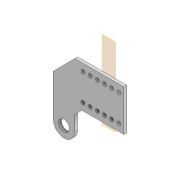
# Autodesk Inventor part: driven wheel arm angled adjustable holes
Saved by Autodesk Inventor 2020 (Build 240168000, 168)
## iProperties
Created: 2020-01-25
Part Number: driven wheel arm angled adjustable holes
Material: Generic
Document SubType Name: Modeling
Designer: ball
Density: 1 g/cm^3
Appearance: Default
Author: ball
Autodesk Inventor part; units mm, degrees
ref_plane "YZ Plane" through (0, 0, 0) normal (1, 0, 0) x (0, 1, 0)
ref_plane "XZ Plane" through (0, 0, 0) normal (0, 1, 0) x (-1, 0, 0)
ref_plane "XY Plane" through (0, 0, 0) normal (0, 0, 1) x (1, 0, 0)
ref_plane "Work Plane1" through (0, 0, 0) normal (0, 0, 1) x (1, 0, 0)
sketch "Sketch1" plane through (0, 0, 0) normal (0, 0, 1) x (1, 0, 0)
  line L0 (11.43, 0) -> (11.43, -63.5) construction
  line L1 (0, 0) -> (11.43, 0) construction
  line L2 (0, 0) -> (0, -63.5) construction
  line L3 (7.44, -34.7378) -> (0, -34.7378) construction
  circle A0 centre (5.715, -31.75) radius 1.7 construction
  line L4 (0, -63.5) -> (11.43, -63.5) construction
  circle A1 centre (5.715, -55.6597) radius 1.7 construction
  line L5 (21.59, -62.0097) -> (-15.6718, -62.0097)
  line L6 (-22.0218, -25.4) -> (21.59, -25.4)
  line L7 (21.59, -25.4) -> (21.59, -62.0097)
  line L8 (18.415, -31.75) -> (-14.605, -31.75) construction
  line L9 (18.923, -55.6597) -> (-14.605, -55.6597) construction
  circle A2 centre (-31.5722, -81.8048) radius 4.826
  arc A3 (-41.0972, -81.8048) -> (-22.0472, -81.8048) centre (-31.5722, -81.8048) ccw
  line L10 (-22.0218, -25.4) -> (-22.0218, -62.0097) construction
  line L11 (-41.0972, -81.8048) -> (-4.0676, -81.8048) construction
  line L12 (-41.0972, -44.6639) -> (-22.0218, -25.4)
  line L13 (-22.0472, -81.8048) -> (-22.0472, -68.3851)
  line L14 (-15.6718, -62.0097) -> (-22.0472, -68.3851)
  line L15 (-15.6718, -62.0097) -> (-6.6556, -62.0097) construction
  line L16 (21.59, -43.7048) -> (-43.6873, -43.7048) construction
  line L17 (21.59, -43.7048) -> (86.8673, -43.7048) construction
  line L18 (-41.0972, -81.8048) -> (-29.4827, -81.8048) construction
  line L19 (-41.0972, -81.8048) -> (-41.0972, -44.6639)
  line L20 (-41.0972, -81.8048) -> (-3.9563, -81.8048) construction
  circle A4 centre (-14.605, -31.75) radius 1.7
  circle A5 centre (-14.605, -55.6597) radius 1.7
  circle A6 centre (-8.255, -55.6597) radius 1.7
  circle A7 centre (-8.255, -31.75) radius 1.7
  circle A8 centre (-1.905, -55.6597) radius 1.7
  circle A9 centre (-1.905, -31.75) radius 1.7
  circle A10 centre (4.445, -55.6597) radius 1.7
  circle A11 centre (4.445, -31.75) radius 1.7
  circle A12 centre (10.795, -55.6597) radius 1.7
  circle A13 centre (10.795, -31.75) radius 1.7
  circle A14 centre (17.145, -55.6597) radius 1.7
  circle A15 centre (17.145, -31.75) radius 1.7
  point P0 (1.905, -31.75)
  point P1 (2.159, -55.6597)
extrude "Extrusion1" add sketch "Sketch1" along normal blind 2.5
body "Solid1"
